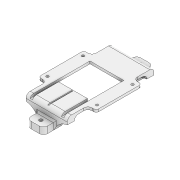
# Autodesk Inventor part: Peltier holder
Saved by Autodesk Inventor 2020 (Build 240168000, 168)
## iProperties
Created: 2020-11-11
Part Number: Peltier holder
Material: Generic
Document SubType Name: Modeling
Designer: ferrerx
Density: 1 g/cm^3
Appearance: White
Author: ferrerx
Autodesk Inventor part; units mm, degrees
ref_plane "YZ Plane" through (0, 0, 0) normal (1, 0, 0) x (0, 1, 0)
ref_plane "XZ Plane" through (0, 0, 0) normal (0, 1, 0) x (-1, 0, 0)
sketch "Sketch1" plane through (0, 0, 0) normal (0, 1, 0) x (-1, 0, 0)
  line L0 (-25, 52.5) -> (25, 52.5)
  line L1 (25, 52.5) -> (25, -52.5)
  line L2 (25, -52.5) -> (-25, -52.5)
  line L3 (-25, -52.5) -> (-25, 52.5)
  line L4 (-25, 52.5) -> (25, -52.5) construction
  line L5 (25, 52.5) -> (-25, -52.5) construction
  circle A0 centre (0, 48.327) radius 1.5
  circle A1 centre (0, -48.237) radius 1.5
  point P0 (0, 0)
  dimension "d0" = 50
  dimension "d1" = 105
  dimension "d2" = 3
  dimension "d3" = 3
  dimension "d4" = 96.564
  dimension "d5" = 48.327
  constraints: 12 end point, 2 centre point, 2 midpoint, 2 parallel, 1 horizontal, 1 perpendicular
  measures "d0" distance of L1.end L2.end
  measures "d1" distance of L2.end L0.start
  measures "d2" diameter of A1
  measures "d3" diameter of A0
  measures "d4" distance of A0.centre A1.centre
  measures "d5" distance of point (0, 0) A0.centre
extrude "Extrusion1" add sketch "Sketch1" along normal blind 3
sketch "Sketch2" plane through (0, 0, 0) normal (0, -1, 0) x (1, 0, 0)
  circle A0 centre (0, 48.327) radius 1.5 projected
  circle A1 centre (0, 48.327) radius 1.5
  circle A2 centre (0, -48.237) radius 1.5 projected
  circle A3 centre (0, -48.237) radius 1.5
  line L0 (-25, 52.5) -> (25, 52.5) projected
  line L1 (25, 52.5) -> (-25, 52.5)
  line L2 (-25, 52.5) -> (-25, 44)
  line L3 (-25, 44) -> (25, 44)
  line L4 (25, 44) -> (25, 52.5)
  line L5 (25, 52.5) -> (25, -52.5) projected
  line L6 (25, -52.5) -> (-25, -52.5)
  line L7 (-25, -52.5) -> (-25, -44)
  line L8 (-25, -44) -> (25, -44)
  line L9 (25, -44) -> (25, -52.5)
  point P0 (0, 0)
  point P1 (25, -44)
  point P2 (-25, 52.5)
  dimension "d9" = 88
  dimension "d50" = 44
  constraints: 16 end point, 4 parallel, 2 centre point, 2 coincident, 2 horizontal, 2 perpendicular
  measures "d9" distance between parallel lines of L8 L3
  measures "d50" distance from line of point (0, 0) L3
extrude "Extrusion2" add sketch "Sketch2" along normal blind 17
sketch "Sketch3" plane through (0, 3, 0) normal (0, 1, 0) x (1, 0, 0)
  line L0 (20.5, -20.5) -> (-20.5, -20.5)
  line L1 (-20.5, -20.5) -> (-20.5, 20.5)
  line L2 (-20.5, 20.5) -> (20.5, 20.5)
  line L3 (20.5, 20.5) -> (20.5, -20.5)
  line L4 (20.5, -20.5) -> (-20.5, 20.5) construction
  line L5 (-20.5, -20.5) -> (20.5, 20.5) construction
  point P0 (0, 0)
  dimension "d14" = 41
  dimension "d15" = 41
  constraints: 12 end point, 2 midpoint, 2 parallel, 1 horizontal, 1 perpendicular
  measures "d14" distance of L0.end L1.end
  measures "d15" distance of L1.end L2.end
extrude "Extrusion3" cut sketch "Sketch3" against normal blind 18.8
sketch "Sketch4" plane through (0, 3, 0) normal (0, 1, 0) x (1, 0, 0)
  line L0 (-20.5, -20.5) -> (-20.5, 20.5) projected
  line L1 (-25, -52.5) -> (25, -52.5) projected
  line L2 (-20.5, -20.5) -> (-17.5, -20.5)
  line L3 (-17.5, -20.5) -> (-17.5, -52.5)
  line L4 (-17.5, -52.5) -> (-20.5, -52.5)
  line L5 (-20.5, -52.5) -> (-20.5, -20.5)
  line L6 (20.5, 20.5) -> (20.5, -20.5) projected
  line L7 (20.5, -20.5) -> (17.5, -20.5)
  line L8 (17.5, -20.5) -> (17.5, -52.5)
  line L9 (17.5, -52.5) -> (20.5, -52.5)
  line L10 (20.5, -52.5) -> (20.5, -20.5)
  point P0 (0, 0)
  dimension "d18" = 3
  dimension "d19" = 3
  constraints: 16 end point, 4 parallel, 2 horizontal, 2 perpendicular, 2 point on line
  measures "d18" distance between parallel lines of L8 L10
  measures "d19" distance between parallel lines of L5 L3
extrude "Extrusion4" cut sketch "Sketch4" against normal blind 3
sketch "Sketch5" plane through (0, -17, 0) normal (0, -1, 0) x (1, 0, 0)
  circle A0 centre (0, 48.327) radius 1.5 projected
  circle A1 centre (0, 48.327) radius 2
  circle A2 centre (0, -48.237) radius 1.5 projected
  circle A3 centre (0, -48.237) radius 2
  point P0 (0, 0)
  dimension "d22" = 4
  dimension "d23" = 4
  constraints: 2 centre point, 2 coincident
  measures "d22" diameter of A1
  measures "d23" diameter of A3
extrude "Extrusion5" cut sketch "Sketch5" against normal blind 5
sketch "Sketch6" plane through (0, 3, 0) normal (0, 1, 0) x (1, 0, 0)
  circle A0 centre (0, 48.237) radius 1.5 projected
  circle A1 centre (0, 48.237) radius 1.5
  circle A2 centre (0, -48.327) radius 1.5 projected
  circle A3 centre (0, -48.327) radius 1.5
  point P0 (0, 0)
  constraints: 2 centre point, 2 coincident
extrude "Extrusion6" add sketch "Sketch6" against normal up to surface (15 mm away)
sketch "Sketch7" plane through (0, 3, 0) normal (0, 1, 0) x (1, 0, 0)
  line L0 (-25, 52.5) -> (-25, -52.5) projected
  line L1 (-25, -27.5) -> (-35, -27.5)
  line L2 (-35, -27.5) -> (-35, 27.5)
  line L3 (-35, 27.5) -> (-25, 27.5)
  line L4 (-25, 27.5) -> (-25, -27.5)
  line L5 (-35, 0) -> (-25, 0) construction
  line L6 (0, 0) -> (-20.5, 0) construction
  line L7 (-20.5, -52.5) -> (-20.5, 20.5) projected
  line L8 (-30, -27.5) -> (-30, 27.5) construction
  circle A0 centre (-30, -21.5) radius 1.55
  circle A1 centre (-30, 21.5) radius 1.55
  line L9 (-17.5, -52.5) -> (17.5, -52.5) projected
  line L10 (0, -52.5) -> (0, 52.5) construction
  line L11 (-25, 52.5) -> (25, 52.5) projected
  line L12 (25, 52.5) -> (25, -52.5)
  line L13 (25, -27.5) -> (35, -27.5)
  line L14 (35, -27.5) -> (35, 27.5)
  line L15 (35, 27.5) -> (25, 27.5)
  line L16 (25, 27.5) -> (25, -27.5)
  line L17 (35, 0) -> (25, 0) construction
  line L18 (20.5, -52.5) -> (20.5, 20.5)
  line L19 (30, -27.5) -> (30, 27.5) construction
  circle A2 centre (30, -21.5) radius 1.55
  circle A3 centre (30, 21.5) radius 1.55
  point P0 (20.5, 0)
  dimension "d28" = 10
  dimension "d29" = 55
  dimension "d30" = 3.1
  dimension "d31" = 3.1
  dimension "d32" = 6
  dimension "d33" = 6
  constraints: 32 end point, 14 symmetric about line, 8 point on line, 6 midpoint, 4 centre point, 2 horizontal, 2 parallel, 1 collinear, 1 perpendicular, 2 other
  measures "d28" distance of L2.end L3.end
  measures "d29" distance of L1.end L2.end
  measures "d30" diameter of A1
  measures "d31" diameter of A0
  measures "d32" distance from line of L3 A1.centre
  measures "d33" distance from line of L1 A0.centre
extrude "Extrusion7" add sketch "Sketch7" against normal blind 3
fillet "Fillet1" radius 3 4 edges at (35, 1.5, -27.5) (35, 1.5, 27.5) (-35, 1.5, -27.5) (-35, 1.5, 27.5)
fillet "Fillet2" radius 5 4 edges at (-25, 1.5, -27.5) (-25, 1.5, 27.5) (25, 1.5, 27.5) (25, 1.5, -27.5)
fillet "Fillet3" radius 5 4 edges at (0, 3, -52.5) (0, 3, 52.5) (-22.75, 3, 52.5) (22.75, 3, 52.5)
fillet "Fillet4" radius 5 4 edges at (0, 0, -44) (0, 0, 44) (-22.75, 0, 44) (22.75, 0, 44)
sketch "Sketch8" plane through (0, 3, 0) normal (0, 1, 0) x (1, 0, 0)
  line L0 (-17.5, -20.5) -> (17.5, -20.5) projected
  line L1 (25, -52.5) -> (-25, -52.5) projected
  line L2 (0.75, -20.5) -> (-0.75, -20.5)
  line L3 (-0.75, -20.5) -> (-0.75, -52.5)
  line L4 (-0.75, -52.5) -> (0.75, -52.5)
  line L5 (0.75, -52.5) -> (0.75, -20.5)
  point P0 (0, 0)
  dimension "d40" = 1.5
  dimension "d41" = 0.75
  constraints: 8 end point, 2 parallel, 2 point on line, 1 horizontal, 1 perpendicular
  measures "d40" distance between parallel lines of L5 L3
  measures "d41" distance from line of L3 point (0, 0)
extrude "Extrusion8" cut sketch "Sketch8" against normal blind 1
fillet "Fillet5" [suppressed]
sketch "Sketch9" plane through (25, -17, -52.5) normal (0, 0, -1) x (-1, 0, 0)
  line L0 (50, 0) -> (0, 0) projected
  arc A0 (15, 0) -> (0, 12) centre (-2.0099, -5.8874) ccw
  line L1 (0, 12) -> (0, 0)
  line L2 (25, 17) -> (25, 0) construction
  line L3 (27, 0) -> (23, 0) projected
  arc A1 (50, 12) -> (35, 0) centre (52.0099, -5.8874) ccw
  line L4 (50, 12) -> (50, 0)
  point P0 (35, 0)
  dimension "d45" = 12
  dimension "d46" = 15
  dimension "d47" = 18
  constraints: 6 end point, 4 point on circle, 3 symmetric about line, 2 centre point, 1 midpoint, 1 point on line, 1 vertical, 1 other
  measures "d45" distance of L1.start L0.end
  measures "d46" distance of L0.end A0.start
  measures "d47" radius of A0
extrude "Extrusion9" cut sketch "Sketch9" against normal blind 116.75
sketch "Sketch10" plane through (0, -17, 0) normal (0, -1, 0) x (1, 0, 0)
  line L0 (-25, 52.5) -> (25, 52.5) projected
  line L1 (10, 52.5) -> (-10, 52.5)
  line L2 (-10, 52.5) -> (-10, 66.5)
  line L3 (-10, 66.5) -> (10, 66.5)
  line L4 (10, 66.5) -> (10, 52.5)
  line L5 (-10, 52.5) -> (-10, 44) projected
  line L6 (0, 66.5) -> (0, 52.5) construction
  circle A0 centre (0, 59.5) radius 2.05
  point P0 (0, 0)
  dimension "d51" = 14
  dimension "d52" = 4.1
  constraints: 10 end point, 3 midpoint, 2 parallel, 1 centre point, 1 collinear, 1 horizontal, 1 perpendicular, 1 point on line
  measures "d51" distance of L1.end L2.end
  measures "d52" diameter of A0
extrude "Extrusion10" add sketch "Sketch10" against normal blind 8
ref_plane "Work Plane1" through (-17.5, 0, 0) normal (0, 0, -1) x (-1, 0, 0)
mirror "Mirror1" about plane through (-17.5, 0, 0) normal (0, 0, -1) of "Extrusion10"
fillet "Fillet6" radius 5 4 edges at (10, -13, 66.5) (-10, -13, 66.5) (10, -13, -66.5) (-10, -13, -66.5)
fillet "Fillet7" radius 2 6 edges at (0, -9, 52.5) (0, -9, -52.5) (10, -13, -52.5) (-10, -13, -52.5) (10, -13, 52.5) (-10, -13, 52.5)
equation "\"d50\" = 0.5 * d9"
body "Solid1"
